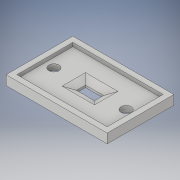
# Autodesk Inventor part: SensorShield
Saved by Autodesk Inventor 2019.3 (Build 233278000, 278)
## iProperties
Created: 2019-04-10
Part Number: SensorShield
Material: Типовые
Document SubType Name: Modeling
Designer: Andrew
Density: 1 g/cm^3
Appearance: По умолчанию
Author: Andrew
## iProperties of the stored document SensorShield_3DПЕЧАТЬ.ipt
Created: 2019-04-10
Part Number: SensorShield_3DПЕЧАТЬ
Material: Типовые
Document SubType Name: Modeling
Designer: Andrew
Density: 1 g/cm^3
Appearance: По умолчанию
Author: Andrew
Autodesk Inventor part; units mm, degrees
ref_plane "YZ Plane" through (0, 0, 0) normal (1, 0, 0) x (0, 1, 0)
ref_plane "XZ Plane" through (0, 0, 0) normal (0, 1, 0) x (-1, 0, 0)
ref_plane "XY Plane" through (0, 0, 0) normal (0, 0, 1) x (1, 0, 0)
sketch "Эскиз1" plane through (0, 0, 0) normal (0, 1, 0) x (-1, 0, 0)
  line L0 (8.9811, 8.3302) -> (-19.0189, 8.3302)
  line L1 (-19.0189, 8.3302) -> (-19.0189, -10.1698)
  line L2 (-19.0189, -10.1698) -> (8.9811, -10.1698)
  line L3 (8.9811, -10.1698) -> (8.9811, 8.3302)
  point P0 (0, 0)
  dimension "d0" = 28
  dimension "d1" = 18.5
  constraints: 8 end point, 2 parallel, 1 horizontal, 1 perpendicular
  measures "d0" distance of L1.end L2.end
  measures "d1" distance of L2.end L0.start
extrude "Выдавливание1" add sketch "Эскиз1" along normal blind 1.6
sketch "Эскиз2" plane through (0, 1.6, 0) normal (0, 1, 0) x (1, 0, 0)
  line L0 (-8.9811, -8.3302) -> (19.0189, -8.3302) projected
  line L1 (19.0189, -8.3302) -> (19.0189, 10.1698) projected
  line L2 (19.0189, 10.1698) -> (-8.9811, 10.1698) projected
  line L3 (-8.9811, 10.1698) -> (-8.9811, -8.3302) projected
  line L4 (-7.4811, -6.8302) -> (17.5189, -6.8302)
  line L5 (17.5189, -6.8302) -> (17.5189, 8.6698)
  line L6 (17.5189, 8.6698) -> (-7.4811, 8.6698)
  line L7 (-7.4811, 8.6698) -> (-7.4811, -6.8302)
  point P0 (0, 0)
  dimension "d4" = 1.5
  constraints: 8 end point, 3 other
  measures "d4" distance between parallel lines of L3 L7
extrude "Выдавливание2" add sketch "Эскиз2" along normal blind 1
sketch "Эскиз3" plane through (0, 1.6, 0) normal (0, 1, 0) x (1, 0, 0)
  line L0 (2.5189, -0.3302) -> (7.5189, -0.3302)
  line L1 (7.5189, -0.3302) -> (7.5189, 2.1698)
  line L2 (7.5189, 2.1698) -> (2.5189, 2.1698)
  line L3 (2.5189, 2.1698) -> (2.5189, -0.3302)
  line L4 (-7.4811, 8.6698) -> (-7.4811, -6.8302) construction
  line L5 (-7.4811, -6.8302) -> (17.5189, -6.8302) construction
  line L6 (17.5189, -6.8302) -> (17.5189, 8.6698) construction
  line L7 (17.5189, 8.6698) -> (-7.4811, 8.6698) construction
  line L8 (5.0189, -0.3302) -> (5.0189, -6.8302) construction
  line L9 (5.0189, 2.1698) -> (5.0189, 8.6698) construction
  line L10 (-7.4811, 0.9198) -> (2.5189, 0.9198) construction
  line L11 (7.5189, 0.9198) -> (17.5189, 0.9198) construction
  point P0 (0, 0)
  dimension "d7" = 5
  dimension "d8" = 2.5
  constraints: 16 end point, 8 midpoint, 2 collinear, 2 parallel, 2 perpendicular, 1 horizontal, 1 point on line
  measures "d7" distance of L1.end L2.end
  measures "d8" distance of L2.end L0.start
extrude "Выдавливание3" cut sketch "Эскиз3" against normal through all
chamfer "Фаска1" distance 2 distance2 1 1 edges at (5.0189, 1.6, -2.1698) measured on face at (5.8522, 1.6, -6.5031)
chamfer "Фаска2" distance 2 distance2 1 1 edges at (2.5189, 1.6, -0.9198) measured on face at (5.8522, 1.6, 4.6635)
chamfer "Фаска3" distance 2 distance2 1 1 edges at (5.0189, 1.6, 0.3302) measured on face at (5.8522, 1.6, 4.6635)
chamfer "Фаска4" distance 2 distance2 1 1 edges at (7.5189, 1.6, -0.9198) measured on face at (14.1855, 1.6, -0.5031)
sketch "Эскиз4" plane through (0, 1.6, 0) normal (0, 1, 0) x (1, 0, 0)
  line L0 (-7.4811, 8.6698) -> (17.5189, 8.6698) projected
  line L1 (-4.9811, 0.9198) -> (-7.4811, 0.9198) construction
  line L2 (15.0189, 0.9198) -> (17.5189, 0.9198) construction
  line L3 (-7.4811, -6.8302) -> (-7.4811, 8.6698) construction
  line L4 (17.5189, 8.6698) -> (17.5189, -6.8302) construction
  point P0 (0, 0)
  dimension "d24" = 20
  constraints: 4 end point, 2 horizontal, 2 midpoint, 1 collinear, 1 horizontal alignment
  measures "d24" distance of L2.start L1.start
hole "Отверстие1" at (15.0189, 1.6, -0.9198) at (-4.9811, 1.6, -0.9198) direction (0, -1, 0) diameter 2.8 end through all
